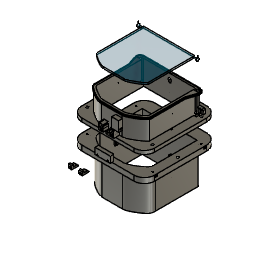
OpenCatFlap (Autodesk Fusion 360 design; units mm, degrees)
Autodesk Fusion 360 part; units mm, degrees
note: some values were not read from the file. Set by a fixed rule: which face or edge a step refers to.
(part 1 of 5)
sketch "Outer_Montage_Rim_1" plane through (0, 0, 0) normal (0, 0, 1) x (1, 0, 0)
  line L0 (30, 0) -> (180, 0)
  line L1 (210, 30) -> (210, 180)
  line L2 (180, 210) -> (30, 210)
  line L3 (0, 180) -> (0, 30)
  arc A0 (30, 210) -> (0, 180) centre (30, 180) ccw
  arc A1 (210, 180) -> (180, 210) centre (180, 180) ccw
  arc A2 (0, 30) -> (30, 0) centre (30, 30) ccw
  arc A3 (180, 0) -> (210, 30) centre (180, 30) ccw
  line L4 (0, 135) -> (21, 135)
  line L5 (210, 135) -> (189, 135)
  line L6 (105, 210) -> (105, 183)
  line L7 (105, 0) -> (105, 11)
  line L8 (105, 11) -> (75, 11)
  line L9 (105, 11) -> (135, 11)
  line L10 (135, 11) -> (290, 11)
  line L11 (189, 135) -> (189, -70)
  line L12 (189, 11) -> (189, 56)
  line L13 (189, 11) -> (189, 36)
  line L14 (189, 36) -> (182, 36)
  spline S0 degree 5 poles (135, 11) (136.1037, 11) (138.5059, 11.2221) (142.694, 12.2217) (149.3091, 14.7818) (158.5187, 19.457) (167.6829, 24.9109) (175.8033, 30.4753) (182.075, 35.6618) (186.0935, 40.3061) (188.1581, 44.7705) (188.7776, 48.7031) (188.9596, 52.1299) (189, 54.6678) (189, 56) knots 0 0 0 0 0 0 0.1 0.2 0.3 0.4 0.5 0.6 0.7 0.8 0.9 1 1 1 1 1 1
  line L15 (130, 11) -> (140, 11)
  line L16 (105, 183) -> (184, 183)
  line L17 (189, 178) -> (189, 135)
  line L18 (21, 135) -> (21, -70)
  spline S1 degree 5 poles (75, 11) (73.8963, 11) (71.4941, 11.2221) (67.306, 12.2217) (60.6909, 14.7818) (51.4813, 19.457) (42.3171, 24.9109) (34.1967, 30.4753) (27.925, 35.6618) (23.9065, 40.3061) (21.8419, 44.7705) (21.2224, 48.7031) (21.0404, 52.1299) (21, 54.6678) (21, 56) knots 0 0 0 0 0 0 0.1 0.2 0.3 0.4 0.5 0.6 0.7 0.8 0.9 1 1 1 1 1 1
  line L19 (189, 46) -> (189, 66)
  line L20 (80, 11) -> (70, 11)
  line L21 (21, 46) -> (21, 66)
  line L22 (105, 11) -> (75, 11)
  arc A4 (189, 178) -> (184, 183) centre (184, 178) ccw
  line L23 (105, 183) -> (26, 183)
  arc A5 (26, 183) -> (21, 178) centre (26, 178) ccw
  line L24 (21, 178) -> (21, 135)
  line L25 (210, 108) -> (199, 108)
  circle A6 centre (199, 108) radius 2
  circle A7 centre (11, 108) radius 2
  line L26 (195.5, 105.9793) -> (199, 103.9585)
  line L27 (199, 103.9585) -> (202.5, 105.9793)
  line L28 (202.5, 105.9793) -> (202.5, 110.0207)
  line L29 (202.5, 110.0207) -> (199, 112.0415)
  line L30 (199, 112.0415) -> (195.5, 110.0207)
  line L31 (195.5, 110.0207) -> (195.5, 105.9793)
  line L32 (11, 103.9585) -> (7.5, 105.9793)
  line L33 (11, 112.0415) -> (14.5, 110.0207)
  line L34 (14.5, 110.0207) -> (14.5, 105.9793)
  circle A8 centre (11, 108) radius 2
  line L35 (14.5, 105.9793) -> (11, 103.9585)
  line L36 (7.5, 105.9793) -> (7.5, 110.0207)
  line L37 (7.5, 110.0207) -> (11, 112.0415)
  point P0 (210, 0)
  point P1 (0, 210)
  point P2 (28, 36)
  point P3 (11, 108)
  point P4 (199, 108)
  point P5 (11, 108)
  point P6 (11, 108)
  dimension "d22" = 210
  dimension "d23" = 210
  dimension "d24" = 30
  dimension "d25" = 30
  dimension "d26" = 30
  dimension "d27" = 30
  dimension "d28" = 21
  dimension "d29" = 21
  dimension "d30" = 27
  dimension "d31" = 11
  dimension "d32" = 30
  dimension "d33" = 30
  dimension "d35" = 45
  dimension "d37" = 25
  dimension "d38" = 7
  dimension "d39" = 5
  dimension "d40" = 11
  dimension "d41" = 4
  dimension "d42" = 108
  dimension "d45" = 3.5
  constraint horizontal L0
  constraint vertical L1
  constraint horizontal L2
  constraint vertical L3
  constraint coincident P1 L2
  constraint coincident P1 L3
  constraint tangent L2 A0
  constraint tangent L3 A0
  constraint tangent L1 A1
  constraint tangent L2 A1
  constraint coincident origin L0
  constraint coincident origin L3
  constraint tangent L0 A2
  constraint tangent L3 A2
  constraint coincident P0 L0
  constraint coincident P0 L1
  constraint tangent L0 A3
  constraint tangent L1 A3
  constraint coincident L3 L4.start
  constraint perpendicular L3 L4
  constraint coincident L1 L5.start
  constraint perpendicular L1 L5
  constraint coincident L2 L6.start
  constraint perpendicular L2 L6
  constraint midpoint L0 L7.start
  constraint perpendicular L0 L7
  constraint perpendicular L7 L8
  constraint perpendicular L7 L9
  constraint parallel L9 L10
  constraint perpendicular L5 L11
  constraint coincident L11 L12.start
  constraint coincident L10 L12.start
  constraint perpendicular L10 L12
  constraint perpendicular L10 L13
  constraint perpendicular L11 L14
  constraint midpoint L9.end L15
  constraint coincident L9 L15.start
  constraint horizontal L16
  constraint vertical L17
  constraint midpoint L12.end L19
  constraint symmetric L5.end L6 L4.end
  constraint symmetric L6 L7.end L8.start
  constraint symmetric L6 L9.end L8.end
  constraint symmetric L6 L11.end L18.end
  constraint symmetric L6 L12.end S1.end
  constraint symmetric L6 L14.end P2
  constraint symmetric L6 L15.start L20.start
  constraint symmetric L6 L15.end L20.end
  constraint symmetric L6 L19.start L21.start
  constraint symmetric L6 L19.end L21.end
  constraint tangent L16 A4
  constraint tangent L17 A4
  constraint midpoint L2 L6.start
  constraint coincident L11 L19.end
  constraint symmetric L16.start L6 L23.start
  constraint symmetric L6 L16.end L23.end
  constraint symmetric L6 L17.start A5.end
  constraint symmetric L6 A4 A5
  constraint coincident L1 L25.start
  constraint perpendicular L1 L25
  constraint coincident P4 L25.end
  constraint symmetric L7 P4 P6
  constraint symmetric L7 A6 A7
  constraint symmetric L7 A6 A8
  constraint symmetric L7 L26.start L34.end
  constraint symmetric L7 L26.end L32.start
  constraint symmetric L7 L27.end L32.end
  constraint symmetric L7 L28.end L36.end
  constraint symmetric L7 L29.end L33.start
  constraint symmetric L7 L30.end L33.end
  measures "d22" distance of origin P0
  measures "d23" distance of origin P1
  measures "d24" radius of A0
  measures "d25" radius of A1
  measures "d26" radius of A2
  measures "d27" radius of A3
  measures "d28" distance of L4.start L4.end
  measures "d29" distance of L5.start L5.end
  measures "d30" distance of L6.start L6.end
  measures "d31" distance of L7.start L7.end
  measures "d32" distance of L7.end L8.end
  measures "d33" distance of L7.end L9.end
  measures "d35" distance of L12.start L12.end
  measures "d37" distance of L12.start L13.end
  measures "d38" distance of L13.end L14.end
  measures "d39" radius of A4
  measures "d40" distance of L25.start P4
  measures "d41" diameter of A6
  measures "d42" distance of L0 L25
  measures "d45" distance of P4 L31
extrude "Extrude1" add sketch "Outer_Montage_Rim_1" along normal blind 10 contours L0 A2 L7 L8 L18 S1 L20 L21 L22 | L0 A3 L7 L9 L10 L11 L15 | L3 A2 L4 L18 L21 | A3 L10 L11 | L2 L3 A0 L4 L6 L23 A5 L24 | L1 A3 L5 L10 L11 L12 L13 L19 | L10 L11 L12 L13 L14 S0 L15 | L11 L12 L14 S0 L19 | L1 L2 A1 L5 L6 L16 L17 A4 | L26 L27 L28 L29 L30 L31 | L32 L33 L34 L35 L36 L37 makes body 1
extrude "Extrude2" cut sketch "Outer_Montage_Rim_1" along normal blind 3.05 from surface at 3 contours L26 L27 L28 L29 L30 L31 | L32 L33 L34 L35 L36 L37 bodies 1
ref_plane "WorkPlane1" through (11, 103.9585, 3) normal (-1, 0, 0) x (0, -1, 0)
sketch "Sketch9" plane through (11, 93.9585, 3) normal (-1, 0, 0) x (0, -1, 0)
  line L0 (-12.0207, 0) -> (-10, 0)
  line L1 (-10, 0) -> (-10, 3.05)
  line L2 (-10, 3.05) -> (-12.0207, 3.05)
  line L3 (-12.0207, 3.05) -> (-12.0207, 0)
  line L4 (-16.0622, 0) -> (-12.0207, 0)
  line L5 (-12.0207, 0) -> (-12.0207, 3.05)
  line L6 (-12.0207, 3.05) -> (-16.0622, 3.05)
  line L7 (-16.0622, 3.05) -> (-16.0622, 0)
  line L8 (-18.0829, 0) -> (-16.0622, 0)
  line L9 (-16.0622, 0) -> (-16.0622, 3.05)
  line L10 (-16.0622, 3.05) -> (-18.0829, 3.05)
  line L11 (-18.0829, 3.05) -> (-18.0829, 0)
  line L12 (-18.0829, 3.05) -> (-10, 3.05)
  line L13 (-10, 3.05) -> (-10, 0)
  line L14 (-10, 0) -> (-18.0829, 0)
  line L15 (-18.0829, 0) -> (-18.0829, 3.05)
  constraint horizontal L12
  constraint vertical L13
  constraint horizontal L14
  constraint vertical L15
  constraint coincident L0.end L1.start
  constraint coincident L10.end L11.start
extrude "Extrude3" cut sketch "Sketch9" against normal blind 188 bodies 1
copy_body "Body->Comp1" bodies 1 removing the originals makes body 2 in component "Outer_Montage_Rim"
sketch "Tunnel" plane through (0, 0, 0) normal (0, 0, 1) x (1, 0, 0)
  line L0 (26, 183) -> (184, 183)
  arc A0 (189, 178) -> (184, 183) centre (184, 178) ccw
  line L1 (189, 178) -> (189, 56)
  spline S0 degree 5 poles (189, 56) (189, 54.6678) (188.9596, 52.1299) (188.7776, 48.7031) (188.1581, 44.7705) (186.0935, 40.3061) (182.075, 35.6618) (175.8033, 30.4753) (167.6829, 24.9109) (158.5187, 19.457) (149.3091, 14.7818) (142.694, 12.2217) (138.5059, 11.2221) (136.1037, 11) (135, 11) knots -1 -1 -1 -1 -1 -1 -0.9 -0.8 -0.7 -0.6 -0.5 -0.4 -0.3 -0.2 -0.1 0 0 0 0 0 0
  line L2 (135, 11) -> (75, 11)
  spline S1 degree 5 poles (75, 11) (73.8963, 11) (71.4941, 11.2221) (67.306, 12.2217) (60.6909, 14.7818) (51.4813, 19.457) (42.3171, 24.9109) (34.1967, 30.4753) (27.925, 35.6618) (23.9065, 40.3061) (21.8419, 44.7705) (21.2224, 48.7031) (21.0404, 52.1299) (21, 54.6678) (21, 56) knots 0 0 0 0 0 0 0.1 0.2 0.3 0.4 0.5 0.6 0.7 0.8 0.9 1 1 1 1 1 1
  line L3 (21, 56) -> (21, 178)
  arc A1 (26, 183) -> (21, 178) centre (26, 178) ccw
  circle A2 centre (11, 108) radius 2
  circle A3 centre (199, 108) radius 2
  arc A4 (180, 0) -> (210, 30) centre (180, 30) ccw
  line L4 (210, 30) -> (210, 180)
  arc A5 (210, 180) -> (180, 210) centre (180, 180) ccw
  line L5 (180, 210) -> (30, 210)
  arc A6 (30, 210) -> (0, 180) centre (30, 180) ccw
  line L6 (0, 180) -> (0, 30)
  arc A7 (0, 30) -> (30, 0) centre (30, 30) ccw
  line L7 (30, 0) -> (180, 0)
  line L8 (135, 13) -> (75, 13)
  spline S2 degree 3 poles (75, 13) (72.879, 13) (69.9606, 13.6226) (66.5308, 14.8436) (61.0368, 16.7995) (54.2498, 20.2368) (47.8772, 24.0253) (43.0977, 26.8667) (38.5778, 29.8827) (34.9301, 32.6852) (31.8875, 35.0228) (29.4648, 37.2071) (27.74, 39.1909) (25.8067, 41.4147) (24.7303, 43.3601) (24.0694, 45.4927) (23.4344, 47.5419) (23.1699, 49.8448) (23.0595, 52.6687) (23.0186, 53.7135) (23, 54.8247) (23, 56) knots 0 0 0 0 0.135002 0.135002 0.135002 0.351252 0.351252 0.351252 0.513439 0.513439 0.513439 0.648723 0.648723 0.648723 0.80037 0.80037 0.80037 0.946083 0.946083 0.946083 1 1 1 1
  line L9 (23, 56) -> (23, 178)
  arc A8 (26, 181) -> (23, 178) centre (26, 178) ccw
  line L10 (26, 181) -> (184, 181)
  arc A9 (187, 178) -> (184, 181) centre (184, 178) ccw
  line L11 (187, 178) -> (187, 56)
  spline S3 degree 3 poles (187, 56) (187, 52.793) (186.8794, 50.0954) (186.481, 47.8125) (186.0053, 45.0874) (185.1528, 42.9091) (183.2655, 40.4245) (181.7979, 38.4924) (179.6595, 36.3812) (176.8375, 34.0823) (173.2701, 31.176) (168.6305, 27.978) (163.6046, 24.917) (158.2458, 21.6532) (152.4827, 18.5707) (147.3855, 16.3874) (143.4879, 14.718) (139.9856, 13.593) (137.2749, 13.1854) (136.4406, 13.06) (135.6806, 13) (135, 13) knots -1 -1 -1 -1 -0.852885 -0.852885 -0.852885 -0.677279 -0.677279 -0.677279 -0.540729 -0.540729 -0.540729 -0.36811 -0.36811 -0.36811 -0.184055 -0.184055 -0.184055 -0.043318 -0.043318 -0.043318 0 0 0 0
  line L12 (135, 16) -> (75, 16)
  spline S4 degree 3 poles (75, 16) (73.6407, 16) (71.4915, 16.3704) (68.8469, 17.2246) (63.8244, 18.8468) (57.0667, 22.1371) (50.6302, 25.8861) (45.8029, 28.6979) (41.1682, 31.7394) (37.4534, 34.5352) (34.6662, 36.633) (32.4058, 38.5922) (30.788, 40.2974) (29.2773, 41.8897) (28.3285, 43.2367) (27.6926, 44.499) (27.0341, 45.806) (26.6597, 47.0839) (26.4026, 48.7672) (26.1107, 50.6784) (26, 53.108) (26, 56) knots 0 0 0 0 0.116327 0.116327 0.116327 0.337245 0.337245 0.337245 0.502934 0.502934 0.502934 0.627254 0.627254 0.627254 0.743338 0.743338 0.743338 0.863534 0.863534 0.863534 1 1 1 1
  line L13 (26, 56) -> (26, 178)
  line L14 (26, 178) -> (184, 178)
  line L15 (184, 178) -> (184, 56)
  spline S5 degree 3 poles (184, 56) (184, 53.3075) (183.9037, 51.0109) (183.6552, 49.1696) (183.4152, 47.3913) (183.0542, 46.0543) (182.4179, 44.7239) (181.7989, 43.4297) (180.8711, 42.0696) (179.3518, 40.4458) (177.5325, 38.5013) (174.8564, 36.2157) (171.5158, 33.7703) (166.6133, 30.1816) (160.3099, 26.2473) (154.1768, 22.9953) (150.0182, 20.7903) (145.9518, 18.9172) (142.5291, 17.6934) (139.736, 16.6948) (137.3746, 16.1501) (135.7618, 16.0299) (135.486, 16.0093) (135.2319, 16) (135, 16) knots -1 -1 -1 -1 -0.872949 -0.872949 -0.872949 -0.750244 -0.750244 -0.750244 -0.630875 -0.630875 -0.630875 -0.48793 -0.48793 -0.48793 -0.278155 -0.278155 -0.278155 -0.135918 -0.135918 -0.135918 -0.019847 -0.019847 -0.019847 0 0 0 0
  dimension "d51" = 2
  dimension "d52" = 5
extrude "Extrude4" add sketch "Tunnel" along normal blind 100 separate body contours L8 S2 L9 A8 L10 A9 L11 S3 makes body 3
sketch "Tunne_end_with_inner_montage" plane through (0, 0, 100) normal (0, 0, 1) x (-1, 0, 0)
  line L0 (-184, -178) -> (-184, -56)
  spline S0 degree 3 poles (-184, -56) (-184, -53.3075) (-183.9037, -51.0109) (-183.6552, -49.1696) (-183.4152, -47.3913) (-183.0542, -46.0543) (-182.4179, -44.7239) (-181.7989, -43.4297) (-180.8711, -42.0696) (-179.3518, -40.4458) (-177.5325, -38.5013) (-174.8564, -36.2157) (-171.5158, -33.7703) (-166.6133, -30.1816) (-160.3099, -26.2473) (-154.1768, -22.9953) (-150.0182, -20.7903) (-145.9518, -18.9172) (-142.5291, -17.6934) (-139.736, -16.6948) (-137.3746, -16.1501) (-135.7618, -16.0299) (-135.486, -16.0093) (-135.2319, -16) (-135, -16) knots -1 -1 -1 -1 -0.872949 -0.872949 -0.872949 -0.750244 -0.750244 -0.750244 -0.630875 -0.630875 -0.630875 -0.48793 -0.48793 -0.48793 -0.278155 -0.278155 -0.278155 -0.135918 -0.135918 -0.135918 -0.019847 -0.019847 -0.019847 0 0 0 0
  line L1 (-135, -16) -> (-75, -16)
  spline S1 degree 3 poles (-75, -16) (-73.6407, -16) (-71.4915, -16.3704) (-68.8469, -17.2246) (-63.8244, -18.8468) (-57.0667, -22.1371) (-50.6302, -25.8861) (-45.8029, -28.6979) (-41.1682, -31.7394) (-37.4534, -34.5352) (-34.6662, -36.633) (-32.4058, -38.5922) (-30.788, -40.2974) (-29.2773, -41.8897) (-28.3285, -43.2367) (-27.6926, -44.499) (-27.0341, -45.806) (-26.6597, -47.0839) (-26.4026, -48.7672) (-26.1107, -50.6784) (-26, -53.108) (-26, -56) knots 0 0 0 0 0.116327 0.116327 0.116327 0.337245 0.337245 0.337245 0.502934 0.502934 0.502934 0.627254 0.627254 0.627254 0.743338 0.743338 0.743338 0.863534 0.863534 0.863534 1 1 1 1
  line L2 (-26, -56) -> (-26, -178)
  line L3 (-26, -178) -> (-184, -178)
  arc A0 (-187, -178) -> (-184, -181) centre (-184, -178) ccw
  line L4 (-184, -181) -> (-26, -181)
  arc A1 (-26, -181) -> (-23, -178) centre (-26, -178) ccw
  line L5 (-23, -178) -> (-23, -56)
  spline S2 degree 3 poles (-23, -56) (-23, -54.8247) (-23.0186, -53.7135) (-23.0595, -52.6687) (-23.1699, -49.8448) (-23.4344, -47.5419) (-24.0694, -45.4927) (-24.7303, -43.3601) (-25.8067, -41.4147) (-27.74, -39.1909) (-29.4648, -37.2071) (-31.8875, -35.0228) (-34.9301, -32.6852) (-38.5778, -29.8827) (-43.0977, -26.8667) (-47.8772, -24.0253) (-54.2498, -20.2368) (-61.0368, -16.7995) (-66.5308, -14.8436) (-69.9606, -13.6226) (-72.879, -13) (-75, -13) knots -1 -1 -1 -1 -0.946083 -0.946083 -0.946083 -0.80037 -0.80037 -0.80037 -0.648723 -0.648723 -0.648723 -0.513439 -0.513439 -0.513439 -0.351252 -0.351252 -0.351252 -0.135002 -0.135002 -0.135002 0 0 0 0
  line L6 (-75, -13) -> (-135, -13)
  spline S3 degree 3 poles (-135, -13) (-135.6806, -13) (-136.4406, -13.06) (-137.2749, -13.1854) (-139.9856, -13.593) (-143.4879, -14.718) (-147.3855, -16.3874) (-152.4827, -18.5707) (-158.2458, -21.6532) (-163.6046, -24.917) (-168.6305, -27.978) (-173.2701, -31.176) (-176.8375, -34.0823) (-179.6595, -36.3812) (-181.7979, -38.4924) (-183.2655, -40.4245) (-185.1528, -42.9091) (-186.0053, -45.0874) (-186.481, -47.8125) (-186.8794, -50.0954) (-187, -52.793) (-187, -56) knots 0 0 0 0 0.043318 0.043318 0.043318 0.184055 0.184055 0.184055 0.36811 0.36811 0.36811 0.540729 0.540729 0.540729 0.677279 0.677279 0.677279 0.852885 0.852885 0.852885 1 1 1 1
  line L7 (-187, -56) -> (-187, -178)
  line L8 (-26, -183) -> (-184, -183)
  arc A2 (-189, -178) -> (-184, -183) centre (-184, -178) ccw
  line L9 (-189, -178) -> (-189, -56)
  spline S4 degree 5 poles (-189, -56) (-189, -54.6678) (-188.9596, -52.1299) (-188.7776, -48.7031) (-188.1581, -44.7705) (-186.0935, -40.3061) (-182.075, -35.6618) (-175.8033, -30.4753) (-167.6829, -24.9109) (-158.5187, -19.457) (-149.3091, -14.7818) (-142.694, -12.2217) (-138.5059, -11.2221) (-136.1037, -11) (-135, -11) knots -1 -1 -1 -1 -1 -1 -0.9 -0.8 -0.7 -0.6 -0.5 -0.4 -0.3 -0.2 -0.1 0 0 0 0 0 0
  line L10 (-135, -11) -> (-75, -11)
  spline S5 degree 5 poles (-75, -11) (-73.8963, -11) (-71.4941, -11.2221) (-67.306, -12.2217) (-60.6909, -14.7818) (-51.4813, -19.457) (-42.3171, -24.9109) (-34.1967, -30.4753) (-27.925, -35.6618) (-23.9065, -40.3061) (-21.8419, -44.7705) (-21.2224, -48.7031) (-21.0404, -52.1299) (-21, -54.6678) (-21, -56) knots 0 0 0 0 0 0 0.1 0.2 0.3 0.4 0.5 0.6 0.7 0.8 0.9 1 1 1 1 1 1
  line L11 (-21, -56) -> (-21, -178)
  arc A3 (-26, -183) -> (-21, -178) centre (-26, -178) ccw
  circle A4 centre (-11, -108) radius 2
  circle A5 centre (-199, -108) radius 2
  arc A6 (-180, 0) -> (-210, -30) centre (-180, -30) ccw
  line L12 (-210, -30) -> (-210, -180)
  arc A7 (-210, -180) -> (-180, -210) centre (-180, -180) ccw
  line L13 (-180, -210) -> (-30, -210)
  arc A8 (-30, -210) -> (0, -180) centre (-30, -180) ccw
  line L14 (0, -180) -> (0, -30)
  arc A9 (0, -30) -> (-30, 0) centre (-30, -30) ccw
  line L15 (-30, 0) -> (-180, 0)
  circle A10 centre (-11, -108) radius 3.5
  circle A11 centre (-199, -108) radius 3.5
  dimension "d61" = 7
  dimension "d62" = 7
  constraint concentric A4 A10
  constraint concentric A5 A11
  measures "d61" diameter of A10
  measures "d62" diameter of A11
extrude "Extrude5" add sketch "Tunne_end_with_inner_montage" along normal blind 15 contours A0 L4 A1 L5 S2 L6 S3 L7 | L8 A2 L9 S4 L10 S5 L11 A3 | A6 L12 A7 L13 A8 L14 A9 L15 | A10 | A11 bodies 3
extrude "Extrude6" cut sketch "Tunne_end_with_inner_montage" along normal blind 7 from surface at 8 contours A10 | A11 bodies 3
fillet "Fillet2" radius 1 14 edges at (105, 178, 0) (184, 117, 0) (172.3477, 34.3862, 0) (105, 16, 0) (37.6516, 34.3865, 0) (26, 117, 0) (23.8787, 180.1213, 0) (105, 181, 0) (186.1213, 180.1213, 0) (187, 117, 0) (174.1423, 31.982, 0) (105, 13, 0) (35.8544, 31.9844, 0) (23, 117, 0) on bodies 3
sketch "Sketch14" plane through (0, 0, 115) normal (0, 0, 1) x (-1, 0, 0)
  line L0 (-184, -117) -> (-184, -102)
  line L1 (-184, -102) -> (-179, -102)
  line L2 (-179, -102) -> (-159.8579, -102) construction
  line L3 (-179, -102) -> (-179, -99)
  line L4 (-180.316, -97.1206) -> (-184, -95.7797)
  line L5 (-179, -97.5996) -> (-156.987, -97.5996) construction
  line L6 (-105, -178) -> (-105, -13.5)
  arc A0 (-179, -99) -> (-180.316, -97.1206) centre (-181, -99) ccw
  circle A1 centre (-11, -108) radius 3.5
  line L7 (-26, -56) -> (-26, -178)
  line L8 (-26, -178) -> (-184, -178)
  line L9 (-184, -178) -> (-184, -56)
  spline S0 degree 3 poles (-184, -56) (-184, -53.3075) (-183.9037, -51.0109) (-183.6552, -49.1696) (-183.4152, -47.3913) (-183.0542, -46.0543) (-182.4179, -44.7239) (-181.7989, -43.4297) (-180.8711, -42.0696) (-179.3518, -40.4458) (-177.5325, -38.5013) (-174.8564, -36.2157) (-171.5158, -33.7703) (-166.6133, -30.1816) (-160.3099, -26.2473) (-154.1768, -22.9953) (-150.0182, -20.7903) (-145.9518, -18.9172) (-142.5291, -17.6934) (-139.736, -16.6948) (-137.3746, -16.1501) (-135.7618, -16.0299) (-135.486, -16.0093) (-135.2319, -16) (-135, -16) knots -1 -1 -1 -1 -0.872949 -0.872949 -0.872949 -0.750244 -0.750244 -0.750244 -0.630875 -0.630875 -0.630875 -0.48793 -0.48793 -0.48793 -0.278155 -0.278155 -0.278155 -0.135918 -0.135918 -0.135918 -0.019847 -0.019847 -0.019847 0 0 0 0
  line L10 (-135, -16) -> (-75, -16)
  spline S1 degree 3 poles (-75, -16) (-73.6407, -16) (-71.4915, -16.3704) (-68.8469, -17.2246) (-63.8244, -18.8468) (-57.0667, -22.1371) (-50.6302, -25.8861) (-45.8029, -28.6979) (-41.1682, -31.7394) (-37.4534, -34.5352) (-34.6662, -36.633) (-32.4058, -38.5922) (-30.788, -40.2974) (-29.2773, -41.8897) (-28.3285, -43.2367) (-27.6926, -44.499) (-27.0341, -45.806) (-26.6597, -47.0839) (-26.4026, -48.7672) (-26.1107, -50.6784) (-26, -53.108) (-26, -56) knots 0 0 0 0 0.116327 0.116327 0.116327 0.337245 0.337245 0.337245 0.502934 0.502934 0.502934 0.627254 0.627254 0.627254 0.743338 0.743338 0.743338 0.863534 0.863534 0.863534 1 1 1 1
  line L11 (-30, 0) -> (-180, 0)
  arc A2 (-180, 0) -> (-210, -30) centre (-180, -30) ccw
  line L12 (-210, -30) -> (-210, -180)
  arc A3 (-210, -180) -> (-180, -210) centre (-180, -180) ccw
  line L13 (-180, -210) -> (-30, -210)
  arc A4 (-30, -210) -> (0, -180) centre (-30, -180) ccw
  line L14 (0, -180) -> (0, -30)
  arc A5 (0, -30) -> (-30, 0) centre (-30, -30) ccw
  line L15 (-184, -56) -> (-184, -53.3075)
  line L16 (-184, -53.3075) -> (-183.9037, -51.0109)
  line L17 (-183.9037, -51.0109) -> (-183.6552, -49.1696)
  line L18 (-183.6552, -49.1696) -> (-183.4152, -47.3913)
  line L19 (-183.4152, -47.3913) -> (-183.0542, -46.0543)
  line L20 (-183.0542, -46.0543) -> (-182.4179, -44.7239)
  line L21 (-182.4179, -44.7239) -> (-181.7989, -43.4297)
  line L22 (-181.7989, -43.4297) -> (-180.8711, -42.0696)
  line L23 (-180.8711, -42.0696) -> (-179.3518, -40.4458)
  line L24 (-179.3518, -40.4458) -> (-177.5325, -38.5013)
  line L25 (-177.5325, -38.5013) -> (-174.8564, -36.2157)
  line L26 (-174.8564, -36.2157) -> (-171.5158, -33.7703)
  line L27 (-171.5158, -33.7703) -> (-166.6133, -30.1816)
  line L28 (-166.6133, -30.1816) -> (-160.3099, -26.2473)
  line L29 (-160.3099, -26.2473) -> (-154.1768, -22.9953)
  line L30 (-154.1768, -22.9953) -> (-150.0182, -20.7903)
  line L31 (-150.0182, -20.7903) -> (-145.9518, -18.9172)
  line L32 (-145.9518, -18.9172) -> (-142.5291, -17.6934)
  line L33 (-142.5291, -17.6934) -> (-139.736, -16.6948)
  line L34 (-139.736, -16.6948) -> (-137.3746, -16.1501)
  line L35 (-137.3746, -16.1501) -> (-135.7618, -16.0299)
  line L36 (-135.7618, -16.0299) -> (-135.486, -16.0093)
  line L37 (-135.486, -16.0093) -> (-135.2319, -16)
  line L38 (-135.2319, -16) -> (-135, -16)
  line L39 (-75, -16) -> (-73.6407, -16)
  line L40 (-73.6407, -16) -> (-71.4915, -16.3704)
  line L41 (-71.4915, -16.3704) -> (-68.8469, -17.2246)
  line L42 (-68.8469, -17.2246) -> (-63.8244, -18.8468)
  line L43 (-63.8244, -18.8468) -> (-57.0667, -22.1371)
  line L44 (-57.0667, -22.1371) -> (-50.6302, -25.8861)
  line L45 (-50.6302, -25.8861) -> (-45.8029, -28.6979)
  line L46 (-45.8029, -28.6979) -> (-41.1682, -31.7394)
  line L47 (-41.1682, -31.7394) -> (-37.4534, -34.5352)
  line L48 (-37.4534, -34.5352) -> (-34.6662, -36.633)
  line L49 (-34.6662, -36.633) -> (-32.4058, -38.5922)
  line L50 (-32.4058, -38.5922) -> (-30.788, -40.2974)
  line L51 (-30.788, -40.2974) -> (-29.2773, -41.8897)
  line L52 (-29.2773, -41.8897) -> (-28.3285, -43.2367)
  line L53 (-28.3285, -43.2367) -> (-27.6926, -44.499)
  line L54 (-27.6926, -44.499) -> (-27.0341, -45.806)
  line L55 (-27.0341, -45.806) -> (-26.6597, -47.0839)
  line L56 (-26.6597, -47.0839) -> (-26.4026, -48.7672)
  line L57 (-26.4026, -48.7672) -> (-26.1107, -50.6784)
  line L58 (-26.1107, -50.6784) -> (-26, -53.108)
  line L59 (-26, -53.108) -> (-26, -56)
  line L60 (-26, -56) -> (-26, -178)
  line L61 (-26, -178) -> (-184, -178)
  line L62 (-184, -178) -> (-184, -56)
  spline S2 degree 3 poles (-184, -56) (-184, -53.3075) (-183.9037, -51.0109) (-183.6552, -49.1696) (-183.4152, -47.3913) (-183.0542, -46.0543) (-182.4179, -44.7239) (-181.7989, -43.4297) (-180.8711, -42.0696) (-179.3518, -40.4458) (-177.5325, -38.5013) (-174.8564, -36.2157) (-171.5158, -33.7703) (-166.6133, -30.1816) (-160.3099, -26.2473) (-154.1768, -22.9953) (-150.0182, -20.7903) (-145.9518, -18.9172) (-142.5291, -17.6934) (-139.736, -16.6948) (-137.3746, -16.1501) (-135.7618, -16.0299) (-135.486, -16.0093) (-135.2319, -16) (-135, -16) knots -1 -1 -1 -1 -0.872949 -0.872949 -0.872949 -0.750244 -0.750244 -0.750244 -0.630875 -0.630875 -0.630875 -0.48793 -0.48793 -0.48793 -0.278155 -0.278155 -0.278155 -0.135918 -0.135918 -0.135918 -0.019847 -0.019847 -0.019847 0 0 0 0
  line L63 (-135, -16) -> (-75, -16)
  spline S3 degree 3 poles (-75, -16) (-73.6407, -16) (-71.4915, -16.3704) (-68.8469, -17.2246) (-63.8244, -18.8468) (-57.0667, -22.1371) (-50.6302, -25.8861) (-45.8029, -28.6979) (-41.1682, -31.7394) (-37.4534, -34.5352) (-34.6662, -36.633) (-32.4058, -38.5922) (-30.788, -40.2974) (-29.2773, -41.8897) (-28.3285, -43.2367) (-27.6926, -44.499) (-27.0341, -45.806) (-26.6597, -47.0839) (-26.4026, -48.7672) (-26.1107, -50.6784) (-26, -53.108) (-26, -56) knots 0 0 0 0 0.116327 0.116327 0.116327 0.337245 0.337245 0.337245 0.502934 0.502934 0.502934 0.627254 0.627254 0.627254 0.743338 0.743338 0.743338 0.863534 0.863534 0.863534 1 1 1 1
  line L64 (-30, 0) -> (-180, 0)
  arc A6 (-180, 0) -> (-210, -30) centre (-180, -30) ccw
  line L65 (-210, -30) -> (-210, -180)
  arc A7 (-210, -180) -> (-180, -210) centre (-180, -180) ccw
  line L66 (-180, -210) -> (-30, -210)
  arc A8 (-30, -210) -> (0, -180) centre (-30, -180) ccw
  line L67 (0, -180) -> (0, -30)
  arc A9 (0, -30) -> (-30, 0) centre (-30, -30) ccw
  line L68 (-184, -102) -> (-180.5, -102)
  line L69 (-180.5, -102) -> (-180.5, -99.2)
  line L70 (-180.5, -99.2) -> (-184, -99.2)
  line L71 (-184, -99.2) -> (-184, -102)
  line L72 (-180.5, -104.8) -> (-184, -104.8)
  line L73 (-180.5, -102) -> (-180.5, -104.8)
  line L74 (-179, -102) -> (-179, -105)
  arc A10 (-180.316, -106.8794) -> (-179, -105) centre (-181, -105) ccw
  line L75 (-180.316, -106.8794) -> (-184, -108.2203)
  arc A11 (-29.684, -97.1206) -> (-31, -99) centre (-29, -99) ccw
  line L76 (-28.6, -104.5) -> (-26, -104.5)
  line L77 (-28.6, -102) -> (-28.6, -104.5)
  line L78 (-26, -102) -> (-29.5, -102)
  line L79 (-29.5, -102) -> (-29.5, -99.2)
  line L80 (-29.5, -99.2) -> (-26, -99.2)
  line L81 (-26, -102) -> (-31, -102)
  line L82 (-29.684, -97.1206) -> (-26, -95.7797)
  line L83 (-31, -102) -> (-31, -99)
  line L84 (-26, -99.2) -> (-26, -102)
  line L85 (-105, -178) -> (-105, -167)
  line L86 (-105, -167) -> (-99, -167)
  line L87 (-105, -167) -> (-111, -167)
  arc A12 (-84.5432, -178) -> (-99, -167) centre (-99, -182) ccw
  arc A13 (-111, -167) -> (-125.4568, -178) centre (-111, -182) ccw
  circle A14 centre (-105, -173) radius 5.5
  line L88 (-29.684, -106.8794) -> (-26, -108.2203)
  arc A15 (-31, -105) -> (-29.684, -106.8794) centre (-29, -105) ccw
  line L89 (-31, -102) -> (-31, -105)
  circle A16 centre (-199, -108) radius 3.5
  circle A17 centre (-11, -108) radius 3.5
  point P0 (-26, -102)
  point P1 (-31, -97.5996)
  dimension "d74" = 5
  dimension "d78" = 160
  dimension "d82" = 2
  dimension "d125" = 3.5
  dimension "d126" = 2.8
  dimension "d127" = 3
  dimension "d139" = 11
  dimension "d140" = 6
  dimension "d141" = 6
  dimension "d142" = 15
  dimension "d143" = 15
  dimension "d154" = 11
  dimension "d155" = 6
  constraint midpoint L0.start L9
  constraint parallel L0 L9
  constraint horizontal L2
  constraint perpendicular L2 L3
  constraint horizontal L5
  constraint coincident L4.end L9
  constraint coincident L5.start L3
  constraint coincident L5.start L4
  constraint tangent L3 A0
  constraint tangent L4 A0
  constraint horizontal L68
  constraint vertical L69
  constraint horizontal L70
  constraint vertical L71
  constraint symmetric L69.start L68 L73.start
  constraint symmetric L69.end L68 L72.start
  constraint symmetric L70.end L68 L72.end
  constraint symmetric L1.end L68 L2.start
  constraint symmetric L4.end L68 L75.end
  constraint symmetric L3.end L68 L74.end
  constraint symmetric L4.start L68 A10.start
  constraint symmetric A0 L68 A10
  constraint symmetric L0.end L6 P0
  constraint symmetric L1.end L6 L81.end
  constraint symmetric L5.start L6 P1
  constraint symmetric L4.end L6 L82.end
  constraint symmetric L6 L3.end A11.end
  constraint symmetric L6 L4.start A11.start
  constraint symmetric L6 A0 A11
  constraint symmetric L6 L68.end L78.end
  constraint symmetric L6 L69.end L79.end
  constraint symmetric L6 L70.end L80.end
  constraint parallel L6 L85
  constraint perpendicular L85 L86
  constraint perpendicular L85 L87
  constraint coincident L61 A12.start
  constraint tangent L86 A12
  constraint coincident L8 A13.end
  constraint tangent L87 A13
  constraint coincident L85 A14.centre
  constraint symmetric L6 L1.end L81.end
  constraint symmetric L6 L74.end A15.start
  constraint symmetric L6 A10.start L88.start
  constraint symmetric L6 A10 A15
  constraint symmetric L6 L75.end L88.end
  measures "d74" distance of L0.end L1.end
  measures "d78" angle of L4 L5
  measures "d82" radius of A0
  measures "d125" distance of L0.end L68.end
  measures "d126" distance of L0.end L70.end
  measures "d127" distance of L1.end L3.end
  measures "d139" distance of L6.start L85.end
  measures "d140" distance of L85.end L86.end
  measures "d141" distance of L85.end L87.end
  measures "d142" radius of A12
  measures "d143" radius of A13
  measures "d154" diameter of A14
  measures "d155" distance of L85.end A14.centre
extrude "Extrude8" add sketch "Sketch14" against normal blind 90 contours L0 L1 L9 L62 L72 L73 L74 A10 L75 | L1 L3 L4 A0 L9 L62 L69 L70 | L7 L60 L76 L77 L78 L81 L88 A15 L89 | L7 L60 A11 L79 L80 L81 L82 L83 bodies 3
sketch "Sketch15" plane through (0, 0, 25) normal (0, 0, -1) x (1, 0, 0)
  line L0 (184, -108.2203) -> (184, -104.8)
  line L1 (181, -103.5) -> (184, -103.5)
  line L2 (184, -103.5) -> (184, -99.5)
  line L3 (184, -99.5) -> (181, -99.5)
  line L4 (181, -99.5) -> (181, -103.5)
  line L5 (28, -104) -> (26, -104)
  line L6 (26, -104) -> (26, -100)
  line L7 (26, -100) -> (28, -100)
  line L8 (28.5, -104) -> (26, -104)
  line L9 (26, -104) -> (26, -100)
  line L10 (26, -100) -> (28.5, -100)
  line L11 (28.5, -100) -> (28.5, -104)
  line L12 (179, -99) -> (179, -105)
  arc A0 (179, -105) -> (180.316, -106.8794) centre (181, -105) ccw
  line L13 (180.316, -106.8794) -> (184, -108.2203)
  line L14 (184, -104.8) -> (180.5, -104.8)
  line L15 (180.5, -104.8) -> (180.5, -99.2)
  line L16 (180.5, -99.2) -> (184, -99.2)
  line L17 (184, -99.2) -> (184, -95.7797)
  line L18 (184, -95.7797) -> (180.316, -97.1206)
  arc A1 (180.316, -97.1206) -> (179, -99) centre (181, -99) ccw
  constraint horizontal L1
  constraint vertical L2
  constraint horizontal L3
  constraint vertical L4
  constraint horizontal L5
  constraint vertical L6
  constraint horizontal L7
  constraint horizontal L8
  constraint vertical L9
  constraint horizontal L10
  constraint vertical L11
revolve "Revolve2" add sketch "Sketch15" angle 90 about axis through (184, 108.2203, 25) along (0, -1, 0) contours L0 L12 A0 L13 L14 L15 L16 L17 L18 A1 | L1 L2 L3 L4 bodies 3
revolve "Revolve1" add 1 faces at (27.228, 97.3668, 25) angle 90 about axis through (26, 99.2, 25) along (0, 1, 0) on bodies 3 bodies 3
copy_body "Body->Comp2" bodies 3 removing the originals makes body 4 in component "Tunnel"
sketch "Sketch23" plane through (179, 0, 0) normal (-1, 0, 0) x (0, -1, 0)
  line L0 (-99, 115) -> (-105, 115)
  line L1 (-105, 115) -> (-105, 25)
  line L2 (-105, 25) -> (-99, 25)
  line L3 (-99, 25) -> (-99, 115)
  circle A0 centre (-102, 35) radius 1.5
  line L4 (-99, 25) -> (-105, 25)
  line L5 (-105, 20) -> (-105, 25)
  line L6 (-105, 20) -> (-99, 20)
  line L7 (-99, 20) -> (-99, 25)
  dimension "d128" = 3
  dimension "d1120" = 10
  measures "d128" diameter of A0
  measures "d1120" distance of L2 A0.centre
extrude "Extrude12" cut sketch "Sketch23" against normal blind 5 contours A0 bodies 4 in component "Tunnel"
extrude "Extrude13" cut sketch "Sketch23" against normal blind 5 from surface at 152 contours A0 bodies 4 in component "Tunnel"
sketch "Sketch30" plane through (0, 0, 115) normal (0, 0, 1) x (-1, 0, 0)
  line L0 (-26, -108.2203) -> (-26, -178)
  line L1 (-26, -178) -> (-184, -178)
  line L2 (-184, -178) -> (-184, -108.2203)
  line L3 (-184, -108.2203) -> (-180.316, -106.8794)
  arc A0 (-180.316, -106.8794) -> (-179, -105) centre (-181, -105) ccw
  line L4 (-179, -105) -> (-179, -99)
  arc A1 (-179, -99) -> (-180.316, -97.1206) centre (-181, -99) ccw
  line L5 (-180.316, -97.1206) -> (-184, -95.7797)
  line L6 (-184, -95.7797) -> (-184, -56)
  spline S0 degree 3 poles (-184, -56) (-184, -53.3075) (-183.9037, -51.0109) (-183.6552, -49.1696) (-183.4152, -47.3913) (-183.0542, -46.0543) (-182.4179, -44.7239) (-181.7989, -43.4297) (-180.8711, -42.0696) (-179.3518, -40.4458) (-177.5325, -38.5013) (-174.8564, -36.2157) (-171.5158, -33.7703) (-166.6133, -30.1816) (-160.3099, -26.2473) (-154.1768, -22.9953) (-150.0182, -20.7903) (-145.9518, -18.9172) (-142.5291, -17.6934) (-139.736, -16.6948) (-137.3746, -16.1501) (-135.7618, -16.0299) (-135.486, -16.0093) (-135.2319, -16) (-135, -16) knots -1 -1 -1 -1 -0.872949 -0.872949 -0.872949 -0.750244 -0.750244 -0.750244 -0.630875 -0.630875 -0.630875 -0.48793 -0.48793 -0.48793 -0.278155 -0.278155 -0.278155 -0.135918 -0.135918 -0.135918 -0.019847 -0.019847 -0.019847 0 0 0 0
  line L7 (-135, -16) -> (-75, -16)
  spline S1 degree 3 poles (-75, -16) (-73.6407, -16) (-71.4915, -16.3704) (-68.8469, -17.2246) (-63.8244, -18.8468) (-57.0667, -22.1371) (-50.6302, -25.8861) (-45.8029, -28.6979) (-41.1682, -31.7394) (-37.4534, -34.5352) (-34.6662, -36.633) (-32.4058, -38.5922) (-30.788, -40.2974) (-29.2773, -41.8897) (-28.3285, -43.2367) (-27.6926, -44.499) (-27.0341, -45.806) (-26.6597, -47.0839) (-26.4026, -48.7672) (-26.1107, -50.6784) (-26, -53.108) (-26, -56) knots 0 0 0 0 0.116327 0.116327 0.116327 0.337245 0.337245 0.337245 0.502934 0.502934 0.502934 0.627254 0.627254 0.627254 0.743338 0.743338 0.743338 0.863534 0.863534 0.863534 1 1 1 1
  line L8 (-26, -56) -> (-26, -95.7797)
  line L9 (-26, -95.7797) -> (-29.684, -97.1206)
  arc A2 (-29.684, -97.1206) -> (-31, -99) centre (-29, -99) ccw
  line L10 (-31, -99) -> (-31, -105)
  line L11 (-26, -104.5) -> (-28.6, -104.5)
  line L12 (-28.6, -104.5) -> (-28.6, -102)
  line L13 (-29.5, -99.2) -> (-26, -99.2)
  line L14 (-184, -99.2) -> (-180.5, -99.2)
  line L15 (-180.5, -99.2) -> (-180.5, -104.8)
  line L16 (-180.5, -104.8) -> (-184, -104.8)
  line L17 (-30, 0) -> (-180, 0)
  arc A3 (-180, 0) -> (-210, -30) centre (-180, -30) ccw
  line L18 (-210, -30) -> (-210, -180)
  arc A4 (-210, -180) -> (-180, -210) centre (-180, -180) ccw
  line L19 (-180, -210) -> (-30, -210)
  arc A5 (-30, -210) -> (0, -180) centre (-30, -180) ccw
  line L20 (0, -180) -> (0, -30)
  arc A6 (0, -30) -> (-30, 0) centre (-30, -30) ccw
  line L21 (-105, -210) -> (-105, 0)
  line L22 (-210, -105) -> (0, -105)
  circle A7 centre (-11, -175) radius 2
  line L23 (-16, -178.5) -> (-7, -178.5)
  line L24 (-7, -171.5) -> (-16, -171.5)
  line L25 (-16, -171.5) -> (-16, -178.5)
  line L26 (-7, -178.5) -> (3.5, -178.5)
  line L27 (3.5, -178.5) -> (3.5, -171.5)
  line L28 (3.5, -171.5) -> (-7, -171.5)
  line L29 (-213.5, -171.5) -> (-203, -171.5)
  line L30 (-213.5, -178.5) -> (-213.5, -171.5)
  line L31 (-203, -171.5) -> (-194, -171.5)
  line L32 (-194, -171.5) -> (-194, -178.5)
  line L33 (-203, -178.5) -> (-213.5, -178.5)
  line L34 (-194, -178.5) -> (-203, -178.5)
  circle A8 centre (-199, -175) radius 2
  line L35 (-16, -38.5) -> (-16, -31.5)
  line L36 (-16, -31.5) -> (-7, -31.5)
  line L37 (3.5, -38.5) -> (-7, -38.5)
  line L38 (-7, -31.5) -> (3.5, -31.5)
  line L39 (3.5, -31.5) -> (3.5, -38.5)
  line L40 (-7, -38.5) -> (-16, -38.5)
  circle A9 centre (-11, -35) radius 2
  circle A10 centre (-199, -35) radius 2
  line L41 (-203, -31.5) -> (-213.5, -31.5)
  line L42 (-194, -31.5) -> (-203, -31.5)
  line L43 (-213.5, -31.5) -> (-213.5, -38.5)
  line L44 (-213.5, -38.5) -> (-203, -38.5)
  line L45 (-203, -38.5) -> (-194, -38.5)
  line L46 (-194, -38.5) -> (-194, -31.5)
  line L47 (-26, -99.2) -> (-26, -104.5)
  arc A11 (-31, -105) -> (-29.684, -106.8794) centre (-29, -105) ccw
  line L48 (-29.684, -106.8794) -> (-26, -108.2203)
  circle A12 centre (-199, -108) radius 3.5
  circle A13 centre (-11, -108) radius 3.5
  line L49 (-28.6, -102) -> (-29.5, -102)
  line L50 (-29.5, -102) -> (-29.5, -99.2)
  line L51 (-184, -104.8) -> (-184, -99.2)
  line L52 (-11, -35) -> (-11, -70)
  line L53 (-11, -175) -> (-11, -140)
  circle A14 centre (-11, -175) radius 2
  line L54 (3.5, -178.5) -> (3.5, -171.5)
  line L55 (3.5, -171.5) -> (-7, -171.5)
  line L56 (-16, -171.5) -> (-16, -178.5)
  line L57 (-7, -171.5) -> (-16, -171.5)
  line L58 (-16, -178.5) -> (-7, -178.5)
  line L59 (-7, -178.5) -> (3.5, -178.5)
  line L60 (-16, -143.5) -> (-7, -143.5)
  line L61 (3.5, -143.5) -> (3.5, -136.5)
  line L62 (-7, -143.5) -> (3.5, -143.5)
  line L63 (3.5, -136.5) -> (-7, -136.5)
  line L64 (-16, -136.5) -> (-16, -143.5)
  line L65 (-16, -136.5) -> (-16, -143.5)
  line L66 (3.5, -143.5) -> (3.5, -136.5)
  circle A15 centre (-11, -140) radius 2
  line L67 (-7, -136.5) -> (-16, -136.5)
  circle A16 centre (-11, -140) radius 2
  line L68 (-7, -143.5) -> (3.5, -143.5)
  line L69 (-16, -143.5) -> (-7, -143.5)
  line L70 (3.5, -136.5) -> (-7, -136.5)
  line L71 (-7, -136.5) -> (-16, -136.5)
  line L72 (3.5, -66.5) -> (3.5, -73.5)
  line L73 (-16, -73.5) -> (-16, -66.5)
  line L74 (3.5, -73.5) -> (-7, -73.5)
  line L75 (-7, -66.5) -> (3.5, -66.5)
  line L76 (-7, -73.5) -> (-16, -73.5)
  line L77 (-16, -66.5) -> (-7, -66.5)
  circle A17 centre (-11, -70) radius 2
  line L78 (-203, -143.5) -> (-213.5, -143.5)
  line L79 (-194, -136.5) -> (-194, -143.5)
  circle A18 centre (-199, -140) radius 2
  line L80 (-213.5, -136.5) -> (-203, -136.5)
  circle A19 centre (-199, -140) radius 2
  line L81 (-213.5, -143.5) -> (-213.5, -136.5)
  line L82 (-194, -143.5) -> (-203, -143.5)
  line L83 (-213.5, -143.5) -> (-213.5, -136.5)
  line L84 (-203, -143.5) -> (-213.5, -143.5)
  line L85 (-194, -143.5) -> (-203, -143.5)
  line L86 (-203, -136.5) -> (-194, -136.5)
  line L87 (-203, -136.5) -> (-194, -136.5)
  line L88 (-213.5, -136.5) -> (-203, -136.5)
  line L89 (-194, -136.5) -> (-194, -143.5)
  line L90 (-203, -66.5) -> (-213.5, -66.5)
  line L91 (-194, -73.5) -> (-194, -66.5)
  line L92 (-194, -66.5) -> (-203, -66.5)
  line L93 (-203, -73.5) -> (-194, -73.5)
  line L94 (-213.5, -73.5) -> (-203, -73.5)
  line L95 (-213.5, -66.5) -> (-213.5, -73.5)
  circle A20 centre (-199, -70) radius 2
  point P0 (-210, -180)
  point P1 (-210, -30)
  point P2 (-180, -30)
  point P3 (-184, -32)
  point P4 (-210, -30)
  point P5 (-11, -175)
  point P6 (0, -145)
  point P7 (-11, -140)
  point P8 (-11, -140)
  point P9 (-11, -70)
  point P10 (-199, -140)
  point P11 (-199, -140)
  point P12 (-210, -145)
  point P13 (-199, -140)
  point P14 (-199, -70)
  point P15 (-199, -70)
  dimension "d188" = 4
  dimension "d190" = 7
  dimension "d205" = 70
  dimension "d206" = 15
  dimension "d861" = 35
  dimension "d862" = 4
  dimension "d863" = 7
  dimension "d864" = 4
  dimension "d865" = 7
  dimension "d866" = 4
  dimension "d867" = 7
  constraint midpoint L19 L21.start
  constraint midpoint L17 L21.end
  constraint midpoint L18 L22.start
  constraint midpoint L20 L22.end
  constraint horizontal L23
  constraint horizontal L24
  constraint vertical L25
  constraint horizontal L26
  constraint vertical L27
  constraint horizontal L28
  constraint symmetric A5.end L21 P0
  constraint symmetric L21 A7 A8
  constraint symmetric L21 L23.start L32.end
  constraint symmetric L21 L23.end L33.start
  constraint symmetric L21 L24.start L29.end
  constraint symmetric L21 L24.end L31.end
  constraint symmetric L21 L26.end L30.start
  constraint symmetric L21 L27.end L29.start
  constraint symmetric L1.end L22 P3
  constraint symmetric P0 L22 P4
  constraint symmetric A4.centre L22 P2
  constraint symmetric L22 A7 A9
  constraint symmetric L22 L23.start L35.end
  constraint symmetric L22 L23.end L36.end
  constraint symmetric L22 L24.start L37.end
  constraint symmetric L22 L24.end L35.start
  constraint symmetric L22 L26.end L38.end
  constraint symmetric L22 L27.end L37.start
  constraint symmetric L22 L29.start L43.end
  constraint symmetric L22 L29.end L44.end
  constraint symmetric L22 P0 P4
  constraint symmetric L22 L32.end L42.start
  constraint symmetric L22 L31.end L45.end
  constraint symmetric L22 L33.start L41.start
  constraint symmetric L22 L30.start L41.end
  constraint symmetric L22 A8 A10
  constraint coincident A9.centre L52.start
  constraint parallel L20 L52
  constraint coincident P5 A7.centre
  constraint perpendicular L24 L53
  constraint horizontal L58
  constraint horizontal L57
  constraint vertical L56
  constraint horizontal L59
  constraint vertical L54
  constraint horizontal L55
  constraint horizontal L60
  constraint horizontal L67
  constraint vertical L64
  constraint horizontal L62
  constraint vertical L61
  constraint horizontal L63
  constraint coincident P8 P7
  constraint horizontal L69
  constraint horizontal L71
  constraint vertical L65
  constraint horizontal L68
  constraint vertical L66
  constraint horizontal L70
  constraint coincident P9 L52.end
  constraint symmetric L21 P9 P15
  constraint symmetric L21 P8 P13
  constraint symmetric L21 P6 P12
  constraint symmetric L21 L64.start L79.start
  constraint symmetric L21 L61.end L80.start
  constraint symmetric L21 L60.end L78.start
  constraint symmetric L21 L60.start L79.end
  constraint symmetric L21 L61.start L78.end
  constraint symmetric L21 L63.end L80.end
  constraint symmetric L21 A15 A19
  constraint symmetric L21 A16 A18
  constraint symmetric L21 L72.end L94.start
  constraint symmetric L21 L72.start L90.end
  constraint symmetric L21 L73.start L91.start
  constraint symmetric L21 L75.start L90.start
  constraint symmetric L21 L73.end L91.end
  constraint symmetric L21 L74.end L93.start
  constraint symmetric L21 A17 A20
  measures "d188" diameter of A7
  measures "d190" distance of L23.start L24.end
  measures "d205" distance of L22 P5
  measures "d206" distance of L0 P5
  measures "d861" distance of P5 P8
  measures "d862" diameter of A14
  measures "d863" distance of L24.end L23.start
  measures "d864" diameter of A15
  measures "d865" distance of L64.start L60.start
  measures "d866" diameter of A16
  measures "d867" distance of L60.start L64.start
extrude "Extrude22" cut sketch "Sketch30" against normal blind 8 contours A7 A14 | A8 | A9 | A10 | A15 A16 | A17 | A18 A19 | A20 bodies 4 in component "Tunnel"
extrude "Extrude23" cut sketch "Sketch30" against normal blind 3.3 from surface at -3 contours L18 L29 L31 L32 L33 L34 | L20 L23 L24 L25 L26 L28 L55 L56 L57 L58 L59 | L20 L60 L62 L63 L64 L65 L67 L68 L69 L70 L71 | L20 L73 L74 L75 L76 L77 | L18 L78 L79 L80 L82 L84 L85 L86 L87 L88 L89 | L20 L35 L36 L37 L38 L40 | L18 L41 L42 L44 L45 L46 | L18 L90 L91 L92 L93 L94 bodies 4 in component "Tunnel"
sketch "Sketch128" plane through (0, 16, 0) normal (0, 1, 0) x (-1, 0, 0)
  line L0 (-135, 1) -> (-75, 1)
  line L1 (-75, 1) -> (-75, 115)
  line L2 (-75, 115) -> (-135, 115)
  line L3 (-135, 115) -> (-135, 1)
  line L4 (-105, 1) -> (-104, 1)
  line L5 (-104, 1) -> (-104, 6)
  line L6 (-104, 6) -> (-106, 6)
  line L7 (-106, 6) -> (-106, 56)
  line L8 (-106, 56) -> (-104, 56)
  line L9 (-104, 56) -> (-104, 6)
  line L10 (-104, 56) -> (-106, 56)
  line L11 (-106, 56) -> (-106, 106)
  line L12 (-106, 106) -> (-104, 106)
  line L13 (-104, 106) -> (-104, 56)
  dimension "d1110" = 1
  dimension "d1111" = 5
  dimension "d1112" = 2
  dimension "d1113" = 50
  dimension "d1114" = 2
  dimension "d1115" = 50
  constraint midpoint L0 L4.start
  constraint parallel L0 L4
  constraint perpendicular L4 L5
  constraint horizontal L6
  constraint vertical L7
  constraint horizontal L8
  constraint vertical L9
  constraint horizontal L10
  constraint vertical L11
  constraint horizontal L12
  constraint vertical L13
  measures "d1110" distance of L4.start L4.end
  measures "d1111" distance of L4.end L5.end
  measures "d1112" distance of L5.end L6.end
  measures "d1113" distance of L5.end L8.end
  measures "d1114" distance of L8.end L7.end
  measures "d1115" distance of L8.end L12.end
extrude "Extrude26" cut sketch "Sketch128" against normal blind 10 contours L6 L7 L8 L9 L10 bodies 4 in component "Tunnel"
sketch "Sketch129" plane through (104, 0, 0) normal (1, 0, 0) x (0, 1, 0)
  line L0 (13, 56) -> (13, 6)
  line L1 (13, 6) -> (16, 6)
  line L2 (16, 6) -> (16, 56)
  line L3 (16, 56) -> (13, 56)
  line L4 (13, 6) -> (13, 56)
  line L5 (13, 56) -> (16, 56)
  line L6 (16, 56) -> (16, 6)
  line L7 (16, 6) -> (13, 6)
  line L8 (30, 100) -> (0, 100)
  line L9 (13, 56) -> (16, 100)
  line L10 (13, 56) -> (16, 56)
  line L11 (16, 100) -> (16, 56)
  constraint coincident L0.start L3.end
  constraint coincident L8 L9.end
  constraint coincident L2.end L3.start
extrude "Extrude27" cut sketch "Sketch129" along normal blind 2 contours L3 L5 L9 L10 L11 bodies 4 in component "Tunnel"
ref_plane "WorkPlane4" through (105, 178, 115) normal (0, 0.707107, 0.707107) x (1, 0, 0)
sketch "Sketch32" plane through (105, 178, 115) normal (0, 0.707107, 0.707107) x (1, 0, 0)
  circle A0 centre (0, 7) radius 4.5
  dimension "d216" = 9
  dimension "d217" = 7
  measures "d216" diameter of A0
  measures "d217" distance of origin A0.centre
extrude "Extrude24" cut sketch "Sketch32" along normal blind 30 draft 2.862 from surface at -12 bodies 4 in component "Tunnel"